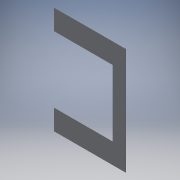
# Autodesk Inventor part: skid plate
Saved by Autodesk Inventor 2016 (Build 200138000, 138)
## iProperties
Created: 2016-02-04
Part Number: skid plate
Material: Aluminum 6061
Document SubType Name: Modeling
Designer: gus
Density: 2.7 g/cm^3
Appearance: Aluminum - Flat
Mass: 514.349 g
Surface Area: 2437.09 cm^2
Volume: 190.5 cm^3
Author: gus
Autodesk Inventor part; units mm, degrees
ref_plane "YZ Plane" through (0, 0, 0) normal (1, 0, 0) x (0, 1, 0)
ref_plane "XZ Plane" through (0, 0, 0) normal (0, 1, 0) x (-1, 0, 0)
ref_plane "XY Plane" through (0, 0, 0) normal (0, 0, 1) x (1, 0, 0)
sketch "Sketch1" plane through (0, 0, 0) normal (0, 0, 1) x (1, 0, 0)
  line L0 (-355.6, 0) -> (-355.6, -101.6)
  line L1 (-355.6, -101.6) -> (0, -101.6)
  line L2 (0, -101.6) -> (0, 0)
  line L3 (-254, 330.2) -> (-355.6, 330.2)
  line L4 (-355.6, 330.2) -> (-355.6, 431.8)
  line L5 (-355.6, 431.8) -> (0, 431.8)
  line L6 (0, 0) -> (0, 431.8)
  line L7 (-355.6, 0) -> (-254, 0)
  line L8 (-254, 330.2) -> (-254, 266.7)
  line L9 (-254, 0) -> (-254, 63.5)
  line L10 (-254, 266.7) -> (-76.2, 266.7)
  line L11 (-76.2, 266.7) -> (-76.2, 63.5)
  line L12 (-76.2, 63.5) -> (-254, 63.5)
  dimension "d4" = 355.6
  dimension "d5" = 101.6
  dimension "d6" = 101.6
  dimension "d7" = 431.8
  dimension "d9" = 63.5
  dimension "d10" = 63.5
  dimension "d11" = 76.2
  dimension "d12" = 101.6
  constraints: 26 end point, 5 perpendicular, 4 vertical, 3 equal length, 3 horizontal, 1 parallel
  measures "d4" distance of L0.end L1.end
  measures "d5" distance of L0.start L0.end
  measures "d6" distance of L1.end L2.end
  measures "d7" distance of L2.end L5.end
  measures "d9" distance of L3.start L8.end
  measures "d10" distance of L7.end L9.end
  measures "d11" distance between parallel lines of L6 L11
  measures "d12" distance between parallel lines of L4 L8
extrude "Extrusion1" add sketch "Sketch1" along normal blind 1.5875
body "Solid1"
